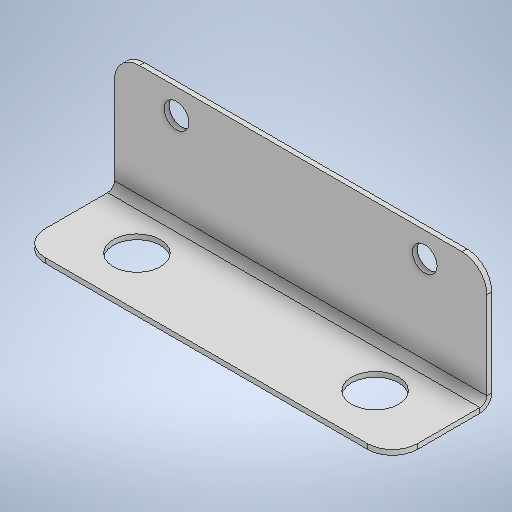
# Autodesk Inventor part: Goat_roller_supp
Saved by Autodesk Inventor 2025 (Build 290162010, 162A)
## iProperties
Created: 2024-09-02
Part Number: Goat_roller_supp
Material: Stainless Steel
Document SubType Name: Sheet Metal
Designer: DELL
Density: 8 g/cm^3
Sheet Metal Rule: AISI304 2mm Die16
Sheet Metal Width: 86,202 mm
Sheet Metal Length: 150,000 mm
Sheet Metal Area: 12930,299 mm^2
Appearance: Default
Flat Pattern Width: 8.6202 cm
Flat Pattern Length: 15 cm
Flat Pattern Area: 129.303 cm^2
Author: DELL
Autodesk Inventor part; units mm, degrees
ref_plane "YZ Plane" through (0, 0, 0) normal (1, 0, 0) x (0, 1, 0)
ref_plane "XZ Plane" through (0, 0, 0) normal (0, 1, 0) x (-1, 0, 0)
ref_plane "XY Plane" through (0, 0, 0) normal (0, 0, 1) x (1, 0, 0)
sketch "Sketch1" plane through (0, 0, 0) normal (0, 0, 1) x (1, 0, 0)
  line L0 (-75, -20) -> (75, -20)
  line L1 (75, -20) -> (75, 20)
  line L2 (75, 20) -> (-75, 20)
  line L3 (-75, 20) -> (-75, -20)
  line L4 (-75, -20) -> (75, 20) construction
  line L5 (75, -20) -> (-75, 20) construction
  circle A0 centre (-48, 0) radius 9.5
  circle A1 centre (48, 0) radius 9.5
  line L6 (0, 20) -> (0, -20) construction
  point P0 (0, 0)
  point P1 (0, 0)
  dimension "d0" = 150
  dimension "d1" = 40
  dimension "d6" = 19
  dimension "d7" = 96
  measures "d0" distance of L2.end L1.end
  measures "d1" distance of L1.end L0.end
  measures "d6" diameter of A0
  measures "d7" distance of A1.centre A0.centre
extrude "Plate1" add sketch "Sketch1" along normal blind 2
sketch "Sketch3" plane through (-75, 18, 0) normal (0, 1, 0) x (-1, 0, 0)
  line L0 (-150, 0) -> (0, 0)
  line L1 (0, 0) -> (0, 50)
  line L2 (0, 50) -> (-150, 50)
  line L3 (-150, 50) -> (-150, 0)
  constraints: 6 end point, 1 horizontal, 1 perpendicular, 1 vertical
edge flange "Flange1" height 50 angle 90 thickness 2 bend radius 2.75 thickness toward (0, 1, 0) relief round relief width 2 relief depth 1 edges at (0, 20, 2) wall of the first edge with corners at (75, 18, 0) (-75, 18, 0) (-75, 18, 50) (75, 18, 50)
bend "Bend1"
corner "Corner1"
sketch "Sketch4" plane through (-75, 20, 50) normal (0, 1, 0) x (1, 0, 0)
  circle A0 centre (25, 10) radius 5
  circle A1 centre (125, 10) radius 5
  line L0 (150, 0) -> (0, 0) construction
  line L1 (75, 0) -> (75, 50) construction
  line L2 (150, 48) -> (0, 48) construction
  dimension "d18" = 10
  dimension "d19" = 10
  dimension "d20" = 100
  constraints: 2 centre point, 2 end point, 1 equal radius, 1 horizontal alignment, 1 midpoint, 1 perpendicular, 1 other
  measures "d18" diameter of A0
  measures "d19" distance from line of L0 A0.centre
  measures "d20" distance of A1.centre A0.centre
extrude "Cut1" cut sketch "Sketch4" against normal blind 2
fillet "Corner Round1" radius 10 4 edges at (75, 19, 50) (-75, -20, 1) (-75, 19, 50) (75, -20, 1)
equation "\"d21\" = Thickness"
equation "\"d2\" = Thickness"
equation "\"d8\" = BendReliefWidth"
equation "\"d9\" = BendReliefDepth"
equation "\"d10\" = MinimumRemnant"
equation "\"d11\" = TransitionRadius"
equation "\"d14\" = BendRadius"
equation "\"d15\" = CornerReliefSize"
equation "\"d16\" = GapSize"
equation "\"d17\" = JacobiRadiusSize"
equation "\"BendReliefWidth\" = Thickness"
equation "\"BendReliefDepth\" = 0.5 * Thickness"
equation "\"CornerReliefSize\" = 4 * Thickness"
equation "\"MinimumRemnant\" = 2 * Thickness"
equation "\"TransitionRadius\" = BendRadius"
equation "\"JacobiRadiusSize\" = BendRadius"
equation "\"GapSize\" = Thickness"
equation "\"Thickness\" = 2"
equation "\"BendRadius\" = 2.75"
body "Solid1"
